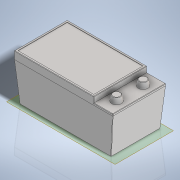
# Autodesk Inventor part: Bateria de camion
Saved by Autodesk Inventor 2022 (Build 260153000, 153)
## iProperties
Created: 2021-09-12
Part Number: Bateria de camion
Material: Generic
Document SubType Name: Modeling
Designer: ARMU
Density: 1 g/cm^3
Appearance: Default
Author: ARMU
Autodesk Inventor part; units mm, degrees
ref_plane "YZ Plane" through (0, 0, 0) normal (1, 0, 0) x (0, 1, 0)
ref_plane "XZ Plane" through (0, 0, 0) normal (0, 1, 0) x (-1, 0, 0)
ref_plane "XY Plane" through (0, 0, 0) normal (0, 0, 1) x (1, 0, 0)
sketch "Sketch1" plane through (0, 0, 0) normal (0, 1, 0) x (-1, 0, 0)
  line L0 (-260, 140) -> (260, 140)
  line L1 (260, 140) -> (260, -140)
  line L2 (260, -140) -> (-260, -140)
  line L3 (-260, -140) -> (-260, 140)
  line L4 (-260, 140) -> (260, -140) construction
  line L5 (260, 140) -> (-260, -140) construction
  point P0 (0, 0)
  dimension "d0" = 520
  dimension "d1" = 280
  constraints: 12 end point, 2 midpoint, 2 parallel, 1 horizontal, 1 perpendicular
  measures "d0" distance of L1.end L2.end
  measures "d1" distance of L0.end L1.end
extrude "Extrusion1" add sketch "Sketch1" along normal blind 40
ref_plane "Work Plane1" through (0, -200, 0) normal (0, -1, 0) x (1, 0, 0)
sketch "Sketch2" plane through (0, -200, 0) normal (0, -1, 0) x (1, 0, 0)
  line L0 (260, -140) -> (-260, -140) construction
  line L1 (-260, 140) -> (260, 140) construction
  line L2 (-260, -140) -> (260, 140) construction
  line L3 (-260, -140) -> (-260, 140) construction
  line L4 (-260, 140) -> (260, -140) construction
  line L5 (-240.6248, 129.5672) -> (240.6248, 129.5672)
  line L6 (240.6248, 129.5672) -> (240.6248, -129.5672)
  line L7 (240.6248, -129.5672) -> (-240.6248, -129.5672)
  line L8 (-240.6248, -129.5672) -> (-240.6248, 129.5672)
  line L9 (-240.6248, 129.5672) -> (240.6248, -129.5672) construction
  line L10 (240.6248, 129.5672) -> (-240.6248, -129.5672) construction
  point P0 (0, 0)
  constraints: 16 end point, 2 midpoint, 2 parallel, 1 horizontal, 1 perpendicular, 1 point on line
loft "Loft1" add profiles "Sketch2" section 2 edges at (0, 0, -140) (260, 0, 0) (0, 0, 140) (-260, 0, 0)
sketch "Sketch3" plane through (0, 40, 0) normal (0, 1, 0) x (1, 0, 0)
  line L0 (260, 140) -> (-260, 140) projected
  line L1 (260, 140) -> (160, 140)
  line L2 (160, 140) -> (160, -140)
  line L3 (160, -140) -> (260, -140)
  line L4 (260, -140) -> (260, 140)
  point P0 (0, 0)
  dimension "d9" = 100
  dimension "d10" = 280
  constraints: 8 end point, 2 parallel, 1 horizontal, 1 perpendicular
  measures "d9" distance of L3.end L2.end
  measures "d10" distance of L2.end L1.end
extrude "Extrusion2" cut sketch "Sketch3" against normal blind 30
sketch "Sketch4" plane through (0, 40, 0) normal (0, 1, 0) x (1, 0, 0)
  line L0 (260, -140) -> (260, 140) construction
  line L1 (260, 140) -> (160, 0) construction
  line L2 (160, -140) -> (160, 140) construction
  line L3 (260, 140) -> (-260, 140) construction
  line L4 (160, 140) -> (260, 0) construction
  line L5 (260, 0) -> (160, -140) construction
  line L6 (-260, -140) -> (260, -140) construction
  line L7 (160, 0) -> (260, -140) construction
  line L8 (160, -140) -> (160, 140) projected
  circle A0 centre (210, 70) radius 20
  circle A1 centre (210, -70) radius 20
  point P0 (0, 0)
  dimension "d13" = 40
  dimension "d14" = 40
  constraints: 8 end point, 4 midpoint, 3 point on line, 2 centre point, 2 parallel
  measures "d13" diameter of A0
  measures "d14" diameter of A1
extrude "Extrusion3" add sketch "Sketch4" against normal blind 30 draft 10
chamfer "Chamfer1" distance 2 angle 45 23 edges at (160, 40, 0) (-50, 40, -140) (160, 25, -140) (210, 10, -140) (260, 10, 0) (210, 10, 140) (160, 25, 140) (-50, 40, 140) (-260, 40, 0) (190, 40, -70) (190, 40, 70) (-260, 20, -140) (-260, 20, 140) (-250.3124, -100, 134.7836) (250.3124, -100, 134.7836) (260, 5, 140) (260, 5, -140) (250.3124, -100, -134.7836) (-250.3124, -100, -134.7836) (-240.6248, -200, 0) (0, -200, -129.5672) (240.6248, -200, 0) (0, -200, 129.5672)
sketch "Sketch5" plane through (0, 40, 0) normal (0, 1, 0) x (1, 0, 0)
  line L0 (-250, 130) -> (150, 130)
  line L1 (150, 130) -> (150, -130)
  line L2 (150, -130) -> (-250, -130)
  line L3 (-250, -130) -> (-250, 130)
  line L4 (160, -138) -> (160, 138) projected
  line L5 (-260, 138) -> (-260, -138) projected
  line L6 (158, 140) -> (-258, 140) projected
  line L7 (-258, -140) -> (158, -140) projected
  point P0 (0, 0)
  dimension "d20" = 10
  dimension "d21" = 10
  dimension "d22" = 10
  dimension "d23" = 10
  constraints: 8 end point, 2 parallel, 1 horizontal, 1 perpendicular
  measures "d20" distance between parallel lines of L4 L1
  measures "d21" distance between parallel lines of L5 L3
  measures "d22" distance between parallel lines of L6 L0
  measures "d23" distance between parallel lines of L2 L7
extrude "Extrusion4" cut sketch "Sketch5" against normal blind 2
body "Solid1"
